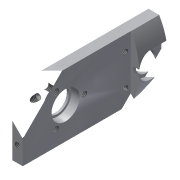
# Autodesk Inventor part: Module Side Beam
Saved by Autodesk Inventor 2014 SP1 (Build 180222100, 222)
## iProperties
Created: 2014-04-22
Part Number: Module Side Beam
Material: Aluminum 6061
Document SubType Name: Modeling
Designer: Rauhul Varma
Density: 2.71 g/cm^3
Appearance: Aluminum - Flat
Mass: 49.0884 g
Surface Area: 77.2953 cm^2
Volume: 18.1138 cm^3
Author: Rauhul Varma
Autodesk Inventor part; units mm, degrees
ref_plane "YZ Plane" through (0, 0, 0) normal (1, 0, 0) x (0, 1, 0)
ref_plane "XZ Plane" through (0, 0, 0) normal (0, 1, 0) x (-1, 0, 0)
ref_plane "XY Plane" through (0, 0, 0) normal (0, 0, 1) x (1, 0, 0)
sketch "Sketch1" plane through (0, 0, 0) normal (0, 0, 1) x (1, 0, 0)
  arc A0 (32.3009, 19.05) -> (32.3009, -19.05) centre (0, 0) ccw construction
  line L0 (0, 0) -> (25.8762, 0) construction
  line L1 (25.8762, 0) -> (25.8762, 19.05)
  line L2 (25.8762, 19.05) -> (32.3009, 19.05)
  line L3 (38.5763, 19.05) -> (38.5763, -19.05) construction
  line L4 (38.5763, -19.05) -> (32.3009, -19.05) construction
  line L5 (25.8762, -19.05) -> (25.8762, 0)
  line L6 (32.3009, 19.05) -> (38.5763, 19.05) construction
  line L7 (32.3009, -19.05) -> (25.8762, -19.05)
  arc A1 (32.3009, -19.05) -> (36.9585, -6.35) centre (0, 0) ccw
  line L8 (30.6388, 19.05) -> (30.6388, -19.05) construction
  line L9 (25.8762, 6.35) -> (36.9585, 6.35) construction
  line L10 (25.8762, -6.35) -> (36.9585, -6.35) construction
  arc A2 (36.9585, 6.35) -> (32.3009, 19.05) centre (0, 0) ccw
  arc A3 (36.9585, -6.35) -> (36.9585, 6.35) centre (0, 0) ccw
  line L11 (36.9585, 6.35) -> (36.9585, -6.35) construction
  point P0 (30.6388, 9.525)
  point P1 (30.6388, -9.525)
  dimension "d0" = 75
  dimension "d1" = 25.8762
  dimension "d2" = 19.05
  dimension "d3" = 19.05
  dimension "d4" = 12.7
  dimension "d5" = 4.7625
  dimension "d6" = 19.05
  dimension "d7" = 9.525
  dimension "d8" = 9.525
  dimension "d9" = 12.7
  dimension "d10" = 6.35
  constraints: 24 end point, 10 point on circle, 6 parallel, 6 perpendicular, 6 point on line, 4 centre point, 1 coincident, 1 collinear, 1 horizontal
  measures "d0" diameter of A0
  measures "d1" distance of L0.start L0.end
  measures "d2" distance of L5.start L0.end
  measures "d3" distance of L0.end L1.end
  measures "d4" distance of L1.end L3.start
  measures "d5" distance between parallel lines of L1 L8
  measures "d6" distance of point (30.639, 9.525) point (30.639, -9.525)
  measures "d7" distance of L8.end point (30.639, -9.525)
  measures "d8" distance of L8.start point (30.639, 9.525)
  measures "d9" distance between parallel lines of L10 L9
  measures "d10" distance between parallel lines of L0 L10
extrude "Extrusion1" add sketch "Sketch1" along normal blind 82.3912
hole "Hole1" at (30.6388, 9.525, 0) at (30.6388, -9.525, 0) direction (0, 0, 1) diameter 3.302 depth 9.525 tip angle 118 thread size "8-32 UNC" class "2B" standard "ANSI Unified Screw Threads"
sketch "Sketch2" plane through (25.8762, -19.05, 0) normal (-1, 0, 0) x (0, 0, 1)
  line L0 (0, 38.1) -> (82.3912, 38.1) projected
  line L1 (0, 19.05) -> (9.525, 19.05) construction
  circle A0 centre (9.525, 19.05) radius 6
  line L2 (82.3912, 38.1) -> (82.3912, 0) projected
  line L3 (9.525, 19.05) -> (56.515, 19.05) construction
  circle A1 centre (56.515, 19.05) radius 8.5
  circle A2 centre (9.525, 19.05) radius 25.4
  circle A3 centre (56.515, 19.05) radius 21.59
  circle A4 centre (56.515, 19.05) radius 7.1437
  dimension "d20" = 9.525
  dimension "d21" = 12
  dimension "d24" = 17
  dimension "d52" = 50.8
  dimension "d53" = 43.18
  dimension "d55" = 14.2875
  constraints: 5 centre point, 5 end point, 4 coincident, 1 parallel, 1 perpendicular, 1 tangent
  measures "d20" distance of L1.start L1.end
  measures "d21" diameter of A0
  measures "d24" diameter of A1
  measures "d52" diameter of A2
  measures "d53" diameter of A3
  measures "d55" diameter of A4
extrude "Extrusion2" cut sketch "Sketch2" against normal through all contours A0 | A4
sketch "Sketch3" plane through (0, 0, 0) normal (0, 0, -1) x (-1, 0, 0)
  line L0 (-25.8762, -19.05) -> (-25.8762, 19.05) projected
  arc A0 (-32.3009, 19.05) -> (-32.3009, -19.05) centre (0, 0) ccw projected
  line L1 (-25.8762, 0) -> (-37.5, 0)
  line L2 (-33.69, 0) -> (-33.69, 7.747)
  line L3 (-33.69, 7.747) -> (-36.6911, 7.747)
  line L4 (-33.69, 0) -> (-33.69, -7.747)
  line L5 (-33.69, -7.747) -> (-36.6911, -7.747)
  line L6 (-37.5, 5.6093) -> (-37.5, -5.6093) construction
  dimension "d28" = 3.81
  dimension "d29" = 15.494
  constraints: 12 end point, 4 perpendicular, 3 point on circle, 1 midpoint, 1 point on line, 1 tangent, 1 vertical, 1 other
  measures "d28" distance between parallel lines of L2 L6
  measures "d29" distance between parallel lines of L5 L3
extrude "Extrusion3" cut sketch "Sketch3" against normal blind 17.272
fillet "Fillet1" radius 7.747 2 edges at (35.1905, -7.747, 17.272) (35.1905, 7.747, 17.272)
sketch "Sketch4" plane through (0, 0, 82.3912) normal (0, 0, 1) x (1, 0, 0)
  line L0 (25.8762, 19.05) -> (25.8762, -19.05) projected
  line L1 (25.8762, -19.05) -> (32.3009, -19.05) projected
  arc A0 (32.3009, -19.05) -> (32.3009, 19.05) centre (0, 0) ccw projected
  line L2 (32.3009, 19.05) -> (25.8762, 19.05) projected
  line L3 (32.2263, 19.05) -> (32.2263, -19.05)
  dimension "d33" = 6.35
  constraints: 2 end point, 2 point on line, 1 perpendicular
  measures "d33" distance between parallel lines of L0 L3
extrude "Extrusion4" cut sketch "Sketch4" against normal blind 65.2475 contours L2 A0 L1 L3
sketch "Sketch5" plane through (32.2263, -19.05, 82.3912) normal (1, 0, 0) x (0, 0, -1)
  line L0 (65.2475, 0) -> (0, 0) projected
  line L1 (65.2475, 0) -> (65.2475, 38.1) projected
  line L2 (0, 38.1) -> (65.2475, 38.1) projected
  line L3 (58.8975, 38.1) -> (58.8975, 0)
  line L4 (62.0725, 38.1) -> (62.0725, 0)
  line L5 (58.8975, 19.05) -> (65.2475, 19.05)
  point P0 (82.3912, 19.05)
  point P1 (62.0725, 28.575)
  point P2 (62.0725, 9.525)
  dimension "d36" = 6.35
  dimension "d37" = 19.05
  dimension "d38" = 9.525
  constraints: 6 end point, 6 point on line, 2 midpoint, 2 perpendicular, 1 other
  measures "d36" distance between parallel lines of L1 L3
  measures "d37" distance of point (62.073, 28.575) point (62.073, 9.525)
  measures "d38" distance from line of L5 point (62.073, 28.575)
hole "Hole2" at (32.2263, 9.525, 20.3187) at (32.2263, -9.525, 20.3187) direction (-1, 0, 0) diameter 3.302 end through all thread size "8-32 UNC" class "2B" standard "ANSI Unified Screw Threads"
extrude "Extrusion6" cut sketch "Sketch2" against normal through all contours A1
extrude "Extrusion7" add sketch "Sketch2" against normal blind 1.35 contours A1
sketch "Sketch7" plane through (0, 0, 82.3912) normal (0, 0, 1) x (1, 0, 0)
  line L0 (32.2263, -19.05) -> (32.2263, 19.05) projected
  line L1 (25.8762, 19.05) -> (25.8762, -19.05) projected
  line L2 (29.0512, 19.05) -> (29.0513, -19.05) construction
  line L3 (25.8762, 0) -> (32.2263, 0) construction
  line L4 (32.2263, 19.05) -> (25.8762, 19.05) projected
  point P0 (0, 0)
  point P1 (29.0513, 9.525)
  point P2 (29.0513, -9.525)
  dimension "d60" = 9.525
  constraints: 4 end point, 3 midpoint, 2 point on line, 1 horizontal alignment, 1 symmetric about line
  measures "d60" distance from line of L3 point (29.051, 9.525)
hole "Hole3" at (29.0513, 9.525, 82.3912) at (29.0513, -9.525, 82.3912) direction (0, 0, -1) diameter 3.302 depth 12.7 tip angle 118 thread size "8-32 UNC" class "2B" standard "ANSI Unified Screw Threads"
sketch "Sketch8" plane through (32.2263, -19.05, 82.3912) normal (1, 0, 0) x (0, 0, -1)
  circle A0 centre (25.8762, 19.05) radius 8.5 projected
  line L0 (0, 38.1) -> (65.2475, 38.1) projected
  circle A1 centre (25.8763, 19.05) radius 11.3766 construction
  line L1 (25.8763, 19.05) -> (37.2528, 19.05) construction
  line L2 (25.8763, 19.05) -> (20.188, 28.9024) construction
  line L3 (25.8763, 19.05) -> (20.188, 9.1976) construction
  circle A2 centre (37.2528, 19.05) radius 3.9688 construction
  circle A3 centre (37.2528, 19.05) radius 2.0828 construction
  point P0 (82.3912, 19.05)
  point P1 (35.17, 19.05)
  point P2 (34.3763, 19.05)
  point P3 (33.2841, 19.05)
  dimension "d70" = 7.9375
  dimension "d71" = 4.1656
  dimension "d68" = 120
  dimension "d69" = 120
  dimension "d72" = 1.0922
  dimension "d73" = 0.7937
  constraints: 6 coincident, 6 end point, 3 horizontal alignment, 3 point on circle, 3 point on line, 1 centre point, 1 parallel, 5 other
  measures "d68" angle of L1 L3
  measures "d69" angle of L1 L2
  measures "d72" distance of point (34.376, 19.05) point (33.284, 19.05)
  measures "d73" distance of point (35.17, 19.05) point (34.376, 19.05)
hole "Hole4" at (32.2263, 0, 45.1384) at (32.2263, -9.8524, 62.2033) at (32.2263, 9.8524, 62.2033) direction (-1, 0, 0) diameter 3.302 end through all thread size "8-32 UNC" class "2B" standard "ANSI Unified Screw Threads"
equation "\"d3\" = d2"
equation "\"d6\" = 2 * d7"
equation "\"d7\" = d8"
body "Solid1"
